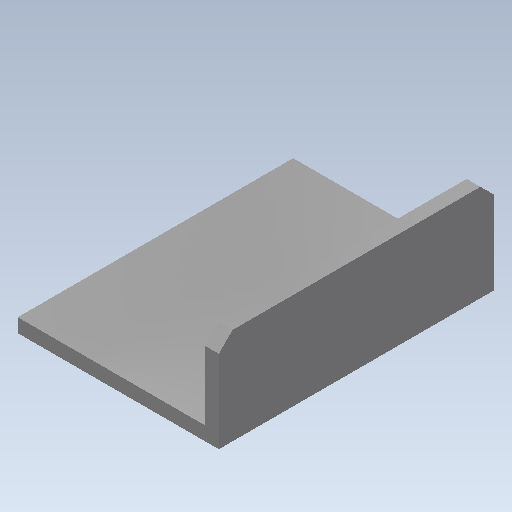
# Autodesk Inventor part: ADSK-MH-10040
Saved by Autodesk Inventor 2020.2 (Build 242310000, 310)
## iProperties
Created: 2008-03-27
Part Number: ADSK-MH-10040
Document SubType Name: Modeling
Designer: R.O'mahony
Density: 7.86 g/cm^3
Mass: 403.808 g
Surface Area: 225.507 cm^2
Volume: 51.375 cm^3
Material: Steel, Mild
Appearance: Steel
Description: Bracket Transfer Support
Engineer: Demir Ali
Checked By: Demir Ali
Company: Autodesk Ltd
Author: R.O'mahony
Keywords: Roller Conveyor
Revision Number: A
Autodesk Inventor part; units mm, degrees
ref_plane "YZ Plane" through (0, 0, 0) normal (1, 0, 0) x (0, 1, 0)
ref_plane "XZ Plane" through (0, 0, 0) normal (0, 1, 0) x (-1, 0, 0)
ref_plane "XY Plane" through (0, 0, 0) normal (0, 0, 1) x (1, 0, 0)
sketch "Sketch1" plane through (0, 0, 0) normal (0, 0, 1) x (1, 0, 0)
  line L0 (2530.6901, -554.9334) -> (2513.6901, -554.9334)
  line L1 (2513.6901, -554.9334) -> (2445.6901, -499.9334)
  line L2 (2518.6901, -464.9334) -> (2518.6901, -499.9334)
  line L3 (2513.6901, -464.9334) -> (2518.6901, -464.9334)
  line L4 (2518.6901, -499.9334) -> (2445.6901, -499.9334)
  line L5 (2445.6901, -499.9334) -> (2445.6901, -494.9334)
  line L6 (2445.6901, -494.9334) -> (2513.6901, -494.9334)
  line L7 (2513.6901, -494.9334) -> (2513.6901, -464.9334)
  line L8 (2523.6901, -464.9334) -> (2535.6901, -505.2758)
  arc A0 (2530.6901, -554.9334) -> (2535.6901, -554.9334) centre (2533.1901, -550.6033) ccw
  line L9 (2523.6901, -464.9334) -> (2518.6901, -464.9334)
  line L10 (2535.6901, -554.9334) -> (2535.6901, -505.2758)
  arc A1 (2530.6901, -554.9334) -> (2535.6901, -554.9334) centre (2533.1901, -550.6033) ccw
  line L11 (2517.6901, -494.9334) -> (1996.6901, -494.9334)
  point P0 (0, 0)
  dimension "d5" = 5
  dimension "d6" = 35
  constraints: 24 end point, 4 point on circle, 2 centre point, 1 collinear
  measures "d5" distance between parallel lines of L6 L4
  measures "d6" distance of L2.start L2.end
extrude "Extrusion1" add sketch "Sketch1" along normal mid plane 100 contours L5 L6 L7 L3 L2 L4
chamfer "Chamfer1" distance 5 angle 45 2 edges at (2516.1901, -464.9334, 50) (2516.1901, -464.9334, -50)
body "Solid1"
